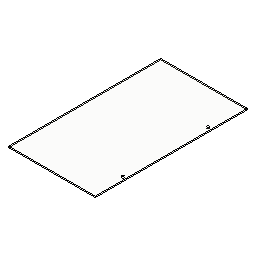
Top Cover v7 (Autodesk Fusion 360 design; units mm, degrees)
Autodesk Fusion 360 part; units mm, degrees
sketch "Sketch1" plane through (0, 0, 0) normal (0, 0, 1) x (1, 0, 0)
  line L0 (0, -50) -> (-137.31, -50)
  line L1 (-137.31, -50) -> (-137.31, 191)
  line L2 (-137.31, 191) -> (0, 191)
  line L3 (0, 191) -> (0, -50)
  dimension "d5" = 137.31
  dimension "d6" = 241
  constraint horizontal L0
  constraint vertical L1
  constraint horizontal L2
  constraint vertical L3
  measures "d5" distance of L0.start L0.end
  measures "d6" distance of L0.start L2.end
extrude "Extrude1" add sketch "Sketch1" along normal blind 2
move_body "Move1" bodies 1 to x (1, 0, 0) y (0, 1, 0) z (0, 0, 1) at (7, 0, 9)
sketch "Sketch2" plane through (0, 0, 11) normal (0, 0, 1) x (-1, 0, 0)
  line L0 (-7, -191) -> (130.31, -191)
  line L1 (130.31, -191) -> (130.31, 50)
  line L2 (130.31, 50) -> (-7, 50)
  line L3 (-7, 50) -> (-7, -191)
  circle A0 centre (-1.05, 0.3) radius 1.6985
sketch "Sketch3" plane through (0, 0, 11) normal (0, 0, 1) x (1, 0, 0)
  circle A0 centre (1.046, 134.9962) radius 1.6656
extrude "Extrude2" cut sketch "Sketch2" sketch "Sketch3" against normal blind 6 contours A0 of sketch 2
